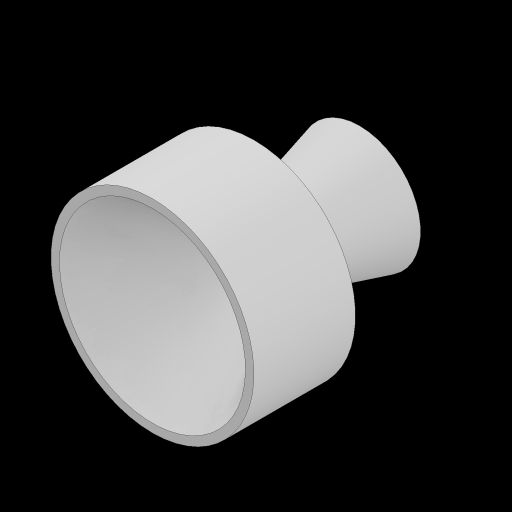
# Autodesk Inventor part: nozzle
Saved by Autodesk Inventor 2023 (Build 270158000, 158)
## iProperties
Created: 2022-11-14
Part Number: nozzle
Material: Generic
Document SubType Name: Modeling
Designer: user
Density: 1 g/cm^3
Appearance: Default
Author: user
Autodesk Inventor part; units mm, degrees
ref_plane "YZ Plane" through (0, 0, 0) normal (1, 0, 0) x (0, 1, 0)
ref_plane "XZ Plane" through (0, 0, 0) normal (0, 1, 0) x (-1, 0, 0)
ref_plane "XY Plane" through (0, 0, 0) normal (0, 0, 1) x (1, 0, 0)
sketch "Sketch1" plane through (0, 0, 0) normal (1, 0, 0) x (0, 1, 0)
  line L0 (22, 22.8504) -> (6, 0)
  line L1 (6, 0) -> (13, -26.1244)
  line L2 (13, -26.1244) -> (14.4343, -26.1244)
  line L3 (14.4343, -26.1244) -> (7.7423, -1.1493)
  line L4 (7.7423, -1.1493) -> (24, -1.1493)
  line L5 (22, 22.8504) -> (24, 22.8504)
  line L6 (24, 22.8504) -> (24, -1.1493)
  line L7 (0, 0) -> (6, 0) construction
  line L8 (0, 0) -> (0, 52.5591) construction
  dimension "d1" = 105
  dimension "d2" = 105
  dimension "d3" = 24
  dimension "d4" = 22
  dimension "d5" = 13
  dimension "d6" = 35
  dimension "d8" = 6
  dimension "d9" = 23.9997
  dimension "d10" = 7.181
  dimension "d11" = 29.7087
  constraints: 18 end point, 3 horizontal, 1 parallel, 1 perpendicular, 1 vertical
  measures "d1" angle of L2 L1
  measures "d2" angle of L2 L3
  measures "d3" distance from line of L7.start L6
  measures "d4" horizontal distance of L7.start L0.start
  measures "d5" horizontal distance of L7.start L1.end
  measures "d6" angle of L8 L0
  measures "d8" distance from line of L8 L0.end
  measures "d9" distance between parallel lines of L5 L4
  measures "d10" distance from line of L7.start L3
  measures "d11" distance from line of L8.end L5
revolve "Revolution1" add sketch "Sketch1" angle 360 about axis through (0, 0, 0) along (0, 0, 1)
body "Solid1"
